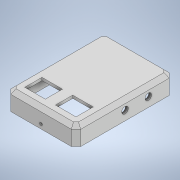
# Autodesk Inventor part: Casing-v2-top
Saved by Autodesk Inventor 2020 (Build 240168000, 168)
## iProperties
Created: 2020-11-25
Part Number: Casing-v2-top
Material: Generic
Document SubType Name: Modeling
Designer: Leon
Density: 1 g/cm^3
Appearance: Default
Author: Leon
Autodesk Inventor part; units mm, degrees
ref_plane "YZ Plane" through (0, 0, 0) normal (1, 0, 0) x (0, 1, 0)
ref_plane "XZ Plane" through (0, 0, 0) normal (0, 1, 0) x (-1, 0, 0)
ref_plane "XY Plane" through (0, 0, 0) normal (0, 0, 1) x (1, 0, 0)
sketch "Sketch5" plane through (0, 0, 0) normal (1, 0, 0) x (0, 1, 0)
  line L0 (10, 52.5) -> (-10, 52.5)
  line L1 (-10, 52.5) -> (-10, -52.5)
  line L2 (-10, -52.5) -> (10, -52.5)
  line L3 (10, -52.5) -> (10, 52.5)
  point P0 (0, 0)
  point P1 (10, 0)
  point P2 (0, -52.5)
  dimension "d6" = 20
  dimension "d30" = 105
  constraints: 8 end point, 2 midpoint, 2 parallel, 1 horizontal, 1 horizontal alignment, 1 perpendicular, 1 vertical alignment
  measures "d6" distance of L0.start L0.end
  measures "d30" distance of L2.end L0.start
extrude "Extrusion2" add sketch "Sketch5" along normal mid plane 75
shell "Shell1" thickness 3 removed faces 1 at (-12.5, -10, 17.5)
chamfer "Chamfer4" distance 5 angle 45 8 edges at (37.5, 0, 52.5) (34.5, -1.5, 49.5) (34.5, -1.5, -49.5) (37.5, 0, -52.5) (-37.5, 0, -52.5) (-34.5, -1.5, -49.5) (-37.5, 0, 52.5) (-34.5, -1.5, 49.5)
sketch "Sketch7" plane through (-37.5, -10, -52.5) normal (0, -1, 0) x (1, 0, 0)
  line L0 (3, 8) -> (3, 97) projected
  line L1 (8, 102) -> (67, 102) projected
  line L2 (72, 97) -> (72, 8) projected
  line L3 (67, 3) -> (8, 3) projected
  line L4 (5, 0) -> (70, 0) projected
  line L5 (75, 100) -> (75, 5) projected
  line L6 (5, 105) -> (70, 105) projected
  line L7 (0, 5) -> (0, 100) projected
  line L8 (8, 102) -> (3, 97) projected
  line L9 (72, 97) -> (67, 102) projected
  line L10 (67, 3) -> (72, 8) projected
  line L11 (3, 8) -> (8, 3) projected
  line L12 (0, 100) -> (5, 105) projected
  line L13 (5, 0) -> (0, 5) projected
  line L14 (75, 5) -> (70, 0) projected
  line L15 (70, 105) -> (75, 100) projected
  line L16 (67.8284, 104) -> (7.1716, 104)
  line L17 (7.1716, 104) -> (1, 97.8284)
  line L18 (1, 97.8284) -> (1, 7.1716)
  line L19 (1, 7.1716) -> (7.1716, 1)
  line L20 (7.1716, 1) -> (67.8284, 1)
  line L21 (67.8284, 1) -> (74, 7.1716)
  line L22 (74, 7.1716) -> (74, 97.8284)
  line L23 (74, 97.8284) -> (67.8284, 104)
  dimension "d61" = 2
  constraints: 16 end point, 7 other
  measures "d61" distance between parallel lines of L9 L23
extrude "Extrusion4" cut sketch "Sketch7" against normal blind 2 contours L23 L22 L21 L20 L19 L18 L17 L16
sketch "Sketch8" plane through (-37.5, 10, 52.5) normal (0, 1, 0) x (1, 0, 0)
  line L0 (32, 10) -> (10, 10)
  line L1 (10, 10) -> (10, 28.5)
  line L2 (10, 28.5) -> (32, 28.5)
  line L3 (32, 28.5) -> (32, 10)
  line L4 (32, 10) -> (10, 28.5) construction
  line L5 (10, 10) -> (32, 28.5) construction
  line L6 (0, 0) -> (0, 105) projected
  line L7 (75, 0) -> (0, 0) projected
  point P0 (37.5, 52.5)
  point P1 (21, 19.25)
  dimension "d35" = 22
  dimension "d36" = 18.5
  dimension "d49" = 10
  dimension "d54" = 10
  constraints: 12 end point, 2 midpoint, 2 parallel, 1 horizontal, 1 perpendicular
  measures "d35" distance of L1.end L2.end
  measures "d36" distance of L0.end L1.end
  measures "d49" distance between parallel lines of L6 L1
  measures "d54" distance between parallel lines of L7 L0
extrude "Extrusion5" cut sketch "Sketch8" against normal blind 3
mirror "Mirror4" about plane through (0, 0, 0) normal (1, 0, 0) of "Extrusion5"
sketch "Sketch9" plane through (37.5, 0, 0) normal (1, 0, 0) x (0, 0, -1)
  circle A0 centre (0, 0) radius 3.5
  circle A1 centre (0, 0) radius 8.5 construction
  line L0 (-8.5, 0) -> (8.5, 0) construction
  line L1 (8.5, 0) -> (8.5, -13) construction
  line L2 (8.5, -13) -> (-8.5, -13) construction
  line L3 (-8.5, -13) -> (-8.5, 0) construction
  dimension "d43" = 17
  dimension "d41" = 7
  dimension "d45" = 13
  dimension "d46" = 0
  constraints: 8 end point, 2 coincident, 2 parallel, 1 centre point, 1 horizontal, 1 horizontal alignment, 1 midpoint, 1 perpendicular, 1 vertical, 2 other
  measures "d41" diameter of A0
  measures "d45" distance of L2.end L0.start
  measures "d46" distance of point (0, 0) A0.centre
extrude "Extrusion6" cut sketch "Sketch9" against normal blind 3
pattern_linear "Rectangular Pattern1" count 2 spacing 25 along (0, 0, -1) of "Extrusion6"
chamfer "Chamfer5" distance 4 angle 45 8 edges at (37.5, 10, 0) (35, 10, 50) (0, 10, 52.5) (-35, 10, 50) (-37.5, 10, 0) (-35, 10, -50) (0, 10, -52.5) (35, 10, -50)
sketch "Sketch10" plane through (32.5, -10, -52.5) normal (0, 0, -1) x (-1, 0, 0)
  line L0 (0, 16) -> (65, 16) projected
  line L1 (0, 0) -> (0, 16) projected
  line L2 (65, 0) -> (0, 0) projected
  line L3 (65, 16) -> (65, 0) projected
  point P0 (32.5, 10)
  point P1 (32.5, 4.75)
  dimension "d65" = 4.75
  constraints: 1 vertical alignment
  measures "d65" distance from line of L2 point (32.5, 4.75)
hole "Hole1" at (0, -5.25, -52.5) direction (0, 0, 1) diameter 3 depth 5
mirror "Mirror5" about plane through (0, 0, 0) normal (0, 0, 1) of "Hole1"
body "Solid2"
